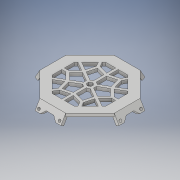
# Autodesk Inventor part: 4-Tool_Lower
Saved by Autodesk Inventor 2019 (Build 230136000, 136)
## iProperties
Created: 2021-01-31
Part Number: 4-Tool_Lower
Material: Generic
Document SubType Name: Modeling
Designer: zhanb
Density: 1 g/cm^3
Appearance: Default
Author: zhanb
Autodesk Inventor part; units mm, degrees
ref_plane "YZ Plane" through (0, 0, 0) normal (1, 0, 0) x (0, 1, 0)
ref_plane "XZ Plane" through (0, 0, 0) normal (0, 1, 0) x (-1, 0, 0)
ref_plane "XY Plane" through (0, 0, 0) normal (0, 0, 1) x (1, 0, 0)
sketch "Sketch1" plane through (0, 0, 0) normal (1, 0, 0) x (0, 1, 0)
  line L0 (76.2, -25.4) -> (50.8, -25.4) construction
  line L1 (50.8, -25.4) -> (50.8, 25.4) construction
  line L2 (50.8, 25.4) -> (76.2, 25.4) construction
  line L3 (76.2, 25.4) -> (76.2, -25.4) construction
  line L4 (76.2, -25.4) -> (50.8, 25.4) construction
  line L5 (50.8, -25.4) -> (76.2, 25.4) construction
  line L6 (76.2, 25.4) -> (-22.7867, 82.55) construction
  line L7 (-22.7867, 82.55) -> (-9.5885, 74.93)
  line L8 (-22.7867, 82.55) -> (-25.9617, 77.0507)
  line L9 (-25.9617, 77.0507) -> (-12.7635, 69.4307)
  line L10 (-9.5885, 74.93) -> (-12.7635, 69.4307) construction
  line L11 (-12.7635, 69.4307) -> (-12.7635, 56.5869)
  line L12 (-12.7635, 56.5869) -> (-6.4135, 56.5869)
  line L13 (-6.4135, 56.5869) -> (-6.4135, 73.0969)
  line L14 (-9.5885, 74.93) -> (-6.4135, 73.0969)
  point P0 (0, 0)
  point P1 (63.5, 0)
  point P2 (-16.1876, 78.74)
  dimension "d0" = 50.8
  dimension "d1" = 25.4
  dimension "d2" = 63.5
  dimension "d3" = 30
  dimension "d4" = 114.3
  dimension "d5" = 15.24
  dimension "d6" = 106.68
  dimension "d7" = 6.35
  dimension "d14" = 6.35
  dimension "d15" = 16.51
  constraints: 30 end point, 6 perpendicular, 3 midpoint, 2 parallel, 2 point on line, 1 collinear, 1 horizontal, 1 horizontal alignment, 1 vertical
  measures "d0" distance of L2.end L0.start
  measures "d1" distance of L1.end L2.end
  measures "d2" distance of point (0, 0) point (63.5, 0)
  measures "d3" angle of L2 L6
  measures "d4" distance of L2.end L6.end
  measures "d5" distance of L6.end L7.end
  measures "d6" distance of L2.end point (-16.188, 78.74)
  measures "d7" distance between parallel lines of L6 L9
  measures "d14" distance of L11.end L12.end
  measures "d15" distance of L13.end L12.end
extrude "Extrusion1" add sketch "Sketch1" along normal mid plane 50.8
pattern_circular "Circular Pattern1" count 4 over 360 about axis through (0, -10, 0) along (0, 1, 0) of "Extrusion1"
sketch "Sketch2" plane through (-25.4, -6.4135, 73.0969) normal (0, 1, 0) x (1, 0, 0)
  line L0 (50.8, 0) -> (0, 0) construction
  line L1 (50.8, 16.51) -> (50.8, 0) construction
  line L2 (50.8, 16.51) -> (0, 16.51) construction
  line L3 (0, 0) -> (0, 16.51) construction
  line L4 (-47.6969, 47.6969) -> (-47.6969, 98.4969) construction
  line L5 (-31.1869, 47.6969) -> (-47.6969, 47.6969) construction
  line L6 (-31.1869, 47.6969) -> (-31.1869, 98.4969) construction
  line L7 (-47.6969, 98.4969) -> (-31.1869, 98.4969) construction
  line L8 (-47.6969, 47.6969) -> (0, 0)
  line L9 (-44.0307, 47.6969) -> (-31.1869, 47.6969) projected
  line L10 (-47.6969, 47.6969) -> (-31.1869, 47.6969)
  line L11 (0, 0) -> (0, 16.51)
  line L12 (0, 3.6662) -> (0, -3.9538) projected
  line L13 (0, 16.51) -> (6.8387, 16.51)
  line L14 (50.8, 16.51) -> (0, 16.51) projected
  line L15 (6.8387, 16.51) -> (-31.1869, 54.5356)
  line L16 (-31.1869, 47.6969) -> (-31.1869, 98.4969) projected
  line L17 (-31.1869, 54.5356) -> (-31.1869, 47.6969)
  point P0 (25.4, 73.0969)
  dimension "d16" = 16.51
  constraints: 12 end point, 2 collinear, 2 point on line, 1 horizontal, 1 parallel
  measures "d16" distance between parallel lines of L15 L8
extrude "Extrusion2" add sketch "Sketch2" against normal up to surface (6.35 mm away)
sketch "Sketch3" plane through (-25.4, -22.7867, 82.55) normal (0, 0.5, 0.8660254) x (1, 0, 0)
  line L0 (50.8, 0) -> (0, 0) construction
  line L1 (10.16, 0) -> (18.034, 7.874)
  line L2 (18.034, 7.874) -> (32.766, 7.874)
  line L3 (32.766, 7.874) -> (40.64, 0)
  line L4 (10.16, 0) -> (40.64, 0)
  line L5 (5.08, 5.08) -> (45.72, 5.08) construction
  line L6 (0, 0) -> (0, 18.9062) construction
  line L7 (50.8, 18.9062) -> (50.8, 0) construction
  point P0 (25.4, 61.0089)
  point P1 (25.4, 7.874)
  point P2 (25.4, 0)
  dimension "d19" = 45
  dimension "d20" = 10.16
  dimension "d21" = 7.874
  dimension "d24" = 5.08
  dimension "d25" = 5.08
  dimension "d26" = 5.08
  constraints: 10 end point, 2 midpoint, 2 parallel, 2 point on line, 1 horizontal, 1 perpendicular, 1 vertical alignment
  measures "d19" angle of L0 L1
  measures "d20" distance of L0.end L1.start
  measures "d21" distance between parallel lines of L0 L2
  measures "d24" distance from line of L0 L5.start
  measures "d25" distance from line of L6 L5.start
  measures "d26" distance from line of L7 L5.end
extrude "Extrusion3" cut sketch "Sketch3" against normal through all
hole "Hole1" at (-20.32, -18.3873, 80.01) at (20.32, -18.3873, 80.01) direction (0, -0.5, -0.8660254) diameter 5.1562 end through all
sketch "Sketch5" plane through (0, 0, 0) normal (1, 0, 0) x (0, 1, 0)
  line L0 (-12.7635, 69.4307) -> (-25.9617, 77.0507) construction
  line L1 (-12.7635, 25.4) -> (-12.7635, 73.0969) projected
  line L2 (-19.1135, 73.0969) -> (-19.1135, 60.3969)
  line L3 (-19.1135, 60.3969) -> (-12.7635, 56.7307)
  line L4 (-12.7635, 69.4307) -> (-12.7635, 56.5869) projected
  line L5 (-12.7635, 69.4307) -> (-19.1135, 73.0969)
  line L6 (-19.1426, 73.1137) -> (-25.9617, 77.0507) projected
  line L7 (-12.7635, 69.4307) -> (-12.7635, 56.7307)
  point P0 (0, 0)
  dimension "d34" = 6.35
  dimension "d35" = 12.7
  constraints: 8 end point, 2 collinear, 2 point on line, 1 parallel, 1 vertical
  measures "d34" distance between parallel lines of L1 L2
  measures "d35" distance of L2.start L2.end
extrude "Extrusion4" add sketch "Sketch5" along normal mid plane 5.08
pattern_circular "Circular Pattern2" count 4 over 360 about axis through (0, -10, 0) along (0, 1, 0) of "Extrusion4", "Extrusion3", "Hole1", "Extrusion2"
sketch "Sketch7" plane through (-25.4, -6.4135, 73.0969) normal (0, 1, 0) x (1, 0, 0)
  line L0 (-47.6969, 47.6969) -> (-47.6969, 98.4969) projected
  line L1 (-47.6969, 47.6969) -> (0, 0) projected
  line L2 (50.8, 0) -> (0, 0) projected
  line L3 (50.8, 0) -> (98.4969, 47.6969) projected
  line L4 (98.4969, 98.4969) -> (98.4969, 47.6969) projected
  line L5 (98.4969, 98.4969) -> (50.8, 146.1938) projected
  line L6 (0, 146.1938) -> (50.8, 146.1938) projected
  line L7 (0, 146.1938) -> (-47.6969, 98.4969) projected
  line L8 (-31.1869, 91.6582) -> (6.8387, 129.6838) projected
  line L9 (6.8387, 129.6838) -> (43.9613, 129.6838) projected
  line L10 (43.9613, 129.6838) -> (81.9869, 91.6582) projected
  line L11 (81.9869, 91.6582) -> (81.9869, 54.5356) projected
  line L12 (81.9869, 54.5356) -> (43.9613, 16.51) projected
  line L13 (43.9613, 16.51) -> (6.8387, 16.51) projected
  line L14 (6.8387, 16.51) -> (-31.1869, 54.5356) projected
  line L15 (-31.1869, 54.5356) -> (-31.1869, 91.6582) projected
  point P0 (25.4, 73.0969)
extrude "Extrusion5" add sketch "Sketch7" against normal up to surface (6.35 mm away) contours L8 L9 L10 L11 L12 L13 L14 L15
sketch "Sketch6" plane through (-25.4, -6.4135, 73.0969) normal (0, 1, 0) x (1, 0, 0)
  line L0 (20.6375, 70.3473) -> (20.6375, 75.8465)
  line L1 (20.6375, 75.8465) -> (25.4, 78.5962)
  line L2 (25.4, 78.5962) -> (30.1625, 75.8465)
  line L3 (30.1625, 75.8465) -> (30.1625, 70.3473)
  line L4 (30.1625, 70.3473) -> (25.4, 67.5977)
  line L5 (25.4, 67.5977) -> (20.6375, 70.3473)
  line L6 (78.1769, 51.236) -> (74.5779, 47.637)
  line L7 (74.5779, 47.637) -> (57.2218, 57.6576)
  line L8 (35.2425, 70.3473) -> (35.2425, 73.0969)
  line L9 (35.2425, 73.0969) -> (65.4769, 73.0969)
  line L10 (78.1769, 73.0969) -> (78.1769, 70.5569) construction
  line L11 (32.7025, 65.9479) -> (50.1272, 55.8877)
  line L12 (70.8591, 43.9182) -> (54.5787, 27.6378)
  line L13 (47.2609, 20.32) -> (27.94, 20.32)
  line L14 (27.94, 20.32) -> (27.94, 37.8188)
  line L15 (27.94, 63.1982) -> (32.7025, 65.9479)
  line L16 (78.1769, 94.9578) -> (78.1769, 51.236) construction
  line L17 (78.1769, 51.236) -> (50.8599, 23.919) construction
  line L18 (47.2609, 20.32) -> (3.5391, 20.32) construction
  line L19 (3.5391, 20.32) -> (-27.3769, 51.236) construction
  line L20 (-27.3769, 51.236) -> (-27.3769, 94.9578) construction
  line L21 (-27.3769, 94.9578) -> (3.5391, 125.8738) construction
  line L22 (3.5391, 125.8738) -> (47.2609, 125.8738) construction
  line L23 (47.2609, 125.8738) -> (78.1769, 94.9578) construction
  line L24 (81.9869, 91.6582) -> (81.9869, 54.5356) construction
  line L25 (30.1625, 70.3473) -> (72.7185, 45.7776) construction
  line L26 (35.2425, 78.7795) -> (35.2425, 67.4143) construction
  line L27 (35.2425, 67.4143) -> (25.4, 61.7318) construction
  line L28 (25.4, 61.7318) -> (15.5575, 67.4143) construction
  line L29 (15.5575, 67.4143) -> (15.5575, 78.7795) construction
  line L30 (15.5575, 78.7795) -> (25.4, 84.4621) construction
  line L31 (25.4, 84.4621) -> (35.2425, 78.7795) construction
  line L32 (78.1769, 70.5569) -> (70.1211, 70.5569)
  line L33 (70.1211, 70.5569) -> (57.2218, 57.6576)
  line L34 (52.6672, 60.2872) -> (65.4769, 73.0969)
  line L35 (65.4769, 73.0969) -> (78.1769, 73.0969) construction
  line L36 (78.1769, 70.5569) -> (78.1769, 51.236)
  line L37 (52.6672, 60.2872) -> (35.2425, 70.3473)
  line L38 (57.2218, 57.6576) -> (52.6672, 60.2872) construction
  line L39 (50.1272, 55.8877) -> (45.4385, 38.3893)
  line L40 (45.4385, 38.3893) -> (27.94, 43.078)
  line L41 (54.6818, 53.2581) -> (49.9603, 35.6373)
  line L42 (49.9603, 35.6373) -> (54.5787, 27.6378)
  line L43 (27.94, 37.8188) -> (45.5609, 33.0973)
  line L44 (45.5609, 33.0973) -> (50.8599, 23.919)
  line L45 (52.7193, 25.7784) -> (30.3213, 64.5731) construction
  line L46 (49.9603, 35.6373) -> (45.4385, 38.3893) construction
  line L47 (45.4385, 38.3893) -> (45.5609, 33.0973) construction
  line L48 (45.5609, 33.0973) -> (49.9603, 35.6373) construction
  line L49 (52.6672, 60.2872) -> (50.1272, 55.8877) construction
  line L50 (50.1272, 55.8877) -> (54.6818, 53.2581) construction
  line L51 (54.6818, 53.2581) -> (70.8591, 43.9182)
  line L52 (27.94, 43.078) -> (27.94, 63.1982)
  line L53 (27.94, 37.8188) -> (27.94, 43.078) construction
  line L54 (54.5787, 27.6378) -> (50.8599, 23.919) construction
  line L55 (50.8599, 23.919) -> (47.2609, 20.32) construction
  line L56 (50.8599, 23.919) -> (47.2609, 20.32)
  point P0 (25.4, 73.0969)
  point P1 (25.4, 73.0969)
  point P2 (25.4, 73.0969)
  point P3 (25.4, 73.0969)
  point P4 (27.7813, 68.9725)
  dimension "d41" = 9.525
  dimension "d42" = 2.54
  dimension "d43" = 5.08
  dimension "d44" = 3.81
  dimension "d45" = 30
  dimension "d46" = 5.08
  dimension "d48" = 5.08
  dimension "d49" = 2.54
  dimension "d50" = 5.08
  dimension "d51" = 5.08
  dimension "d52" = 5.08
  dimension "d61" = 12.7
  constraints: 112 end point, 17 parallel, 12 point on line, 10 collinear, 7 perpendicular, 5 vertical, 4 midpoint, 3 coincident, 3 horizontal, 1 equal length, 46 other
  measures "d41" distance between parallel lines of L0 L3
  measures "d42" distance from line of L4.end L14
  measures "d43" distance between parallel lines of L7 L11
  measures "d44" distance between parallel lines of L24 L16
  measures "d45" angle of L9 L25
  measures "d46" distance between parallel lines of L26 L3
  measures "d48" distance between parallel lines of L34 L33
  measures "d49" distance between parallel lines of L35 L32
  measures "d50" distance between parallel lines of L44 L42
  measures "d51" distance between parallel lines of L39 L41
  measures "d52" distance between parallel lines of L43 L40
  measures "d61" distance of L10.start L9.end
extrude "Extrusion6" cut sketch "Sketch6" against normal through all contours L6 L7 L33 L32 L36 | L8 L9 L34 L37 | L11 L39 L40 L52 L15 | L12 L42 L41 L51 | L13 L14 L43 L44 L56
mirror "Mirror1" about plane through (0, 0, 0) normal (1, 0, 0) of "Extrusion6"
mirror "Mirror2" about plane through (0, 0, 0) normal (0, 0, 1) of "Extrusion6", "Mirror1"
extrude "Extrusion7" cut sketch "Sketch6" against normal through all contours L0 L1 L2 L3 L4 L5
equation "\"d5\" = -2 * d6 + 2 * d4"
equation "\"d26\" = d25"
equation "\"d48\" = d43"
equation "\"d51\" = d50"
equation "\"d52\" = d50"
body "Solid1"
